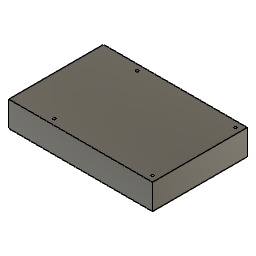
Thermograph (Autodesk Fusion 360 archive; units mm, degrees)
design "Rasp"
Autodesk Fusion 360 part; units mm, degrees
sketch "Skizze1" plane through (0, 0, 0) normal (0, 0, 1) x (1, 0, 0)
  line L0 (0, 0) -> (85, 0)
  line L1 (85, 0) -> (85, 56)
  line L2 (85, 56) -> (0, 56)
  line L3 (0, 56) -> (0, 0)
  dimension "d1" = 85
  dimension "d2" = 56
  constraint horizontal L0
  constraint vertical L1
  constraint horizontal L2
  constraint vertical L3
  constraint coincident L0.start L3.end
  measures "d1" distance of L0.start L0.end
  measures "d2" distance of L0.start L2.end
extrude "Extrusion1" add sketch "Skizze1" along normal blind 15
sketch "Skizze2" plane through (0, 0, 15) normal (0, 0, 1) x (-1, 0, 0)
  line L0 (0, -56) -> (0, 0)
  line L1 (0, 0) -> (-85, 0)
  line L2 (-85, 0) -> (-85, -56)
  line L3 (-85, -56) -> (0, -56)
  point P0 (-23.5, -52.5)
  point P1 (-81.5, -52.5)
  point P2 (-81.5, -3.5)
  point P3 (-23.5, -3.5)
  dimension "d5" = 3.5
  dimension "d6" = 3.5
  dimension "d7" = 3.5
  dimension "d8" = 3.5
  dimension "d9" = 3.5
  dimension "d10" = 3.5
  dimension "d11" = 58
  dimension "d12" = 58
  measures "d5" distance of L2 P2
  measures "d6" distance of L1 P2
  measures "d7" distance of L2 P1
  measures "d8" distance of L3 P1
  measures "d9" distance of L3 P0
  measures "d10" distance of L1 P3
  measures "d11" distance of P0 P1
  measures "d12" distance of P2 P3
hole "Bohrung1" at (23.5, 52.5, 15) at (81.5, 52.5, 15) at (81.5, 3.5, 15) at (23.5, 3.5, 15) direction (0, 0, -1) diameter 1.6 end through all

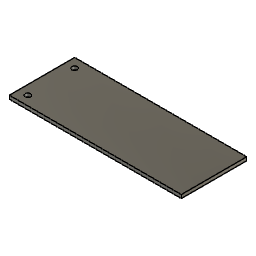
design "MLX"
Autodesk Fusion 360 part; units mm, degrees
sketch "Skizze1" plane through (0, 0, 0) normal (0, 0, 1) x (1, 0, 0)
  line L0 (0, 0) -> (50, 0)
  line L1 (50, 0) -> (50, 19)
  line L2 (50, 19) -> (0, 19)
  line L3 (0, 19) -> (0, 0)
  dimension "d1" = 50
  dimension "d2" = 19
  constraint horizontal L0
  constraint vertical L1
  constraint horizontal L2
  constraint vertical L3
  constraint coincident L0.start L3.end
  measures "d1" distance of L0.start L0.end
  measures "d2" distance of L0.start L2.end
extrude "Extrusion1" add sketch "Skizze1" along normal blind 1
sketch "Skizze2" plane through (0, 0, 1) normal (0, 0, 1) x (-1, 0, 0)
  line L0 (0, -19) -> (0, 0)
  line L1 (0, 0) -> (-50, 0)
  line L2 (-50, 0) -> (-50, -19)
  line L3 (-50, -19) -> (0, -19)
  point P0 (-2.7, -16.3)
  point P1 (-2.7, -2.7)
  dimension "d5" = 2.7
  dimension "d6" = 2.7
  dimension "d7" = 2.7
  dimension "d8" = 2.7
  measures "d5" distance of L0 P0
  measures "d6" distance of L3 P0
  measures "d7" distance of L1 P1
  measures "d8" distance of L0 P1
hole "Bohrung1" at (2.7, 2.7, 1) direction (0, 0, -1) diameter 1.6 depth 3 tip angle 180
hole "Bohrung2" at (2.7, 16.3, 1) direction (0, 0, -1) diameter 1.6 depth 3 tip angle 180

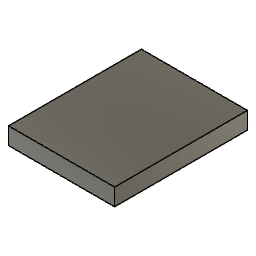
design "akku"
Autodesk Fusion 360 part; units mm, degrees
sketch "Skizze1" plane through (0, 0, 0) normal (0, 0, 1) x (1, 0, 0)
  line L0 (25.15, 31.5) -> (-25.15, 31.5)
  line L1 (-25.15, 31.5) -> (-25.15, -31.5)
  line L2 (-25.15, -31.5) -> (25.15, -31.5)
  line L3 (25.15, -31.5) -> (25.15, 31.5)
  line L4 (25.15, 31.5) -> (-25.15, -31.5) construction
  line L5 (-25.15, 31.5) -> (25.15, -31.5) construction
  dimension "d1" = 63
  dimension "d2" = 50.3
  constraint horizontal L0
  constraint perpendicular L0 L1
  constraint parallel L0 L2
  constraint parallel L1 L3
  constraint coincident L4 origin
  constraint coincident L5 origin
  measures "d1" distance of L0.end L1.end
  measures "d2" distance of L1.end L2.end
extrude "Extrusion1" add sketch "Skizze1" along normal blind 8.1
